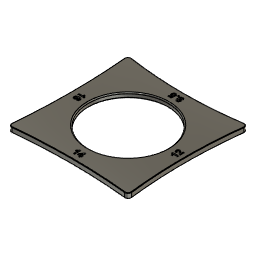
Radius Gauge (Autodesk Fusion 360 design; units mm, degrees)
Autodesk Fusion 360 part; units mm, degrees
note: some values were not read from the file. Set by a fixed rule: which sketch regions a step uses.
sketch "Sketch1" plane through (0, 0, 0) normal (0, 0, 1) x (1, 0, 0)
sketch "Sketch2" plane through (0, 0, 0) normal (0, 0, 1) x (1, 0, 0)
  line L0 (-38.1, 38.1) -> (38.1, 38.1)
  line L1 (38.1, 38.1) -> (38.1, -38.1)
  line L2 (38.1, -38.1) -> (-38.1, -38.1)
  line L3 (-38.1, -38.1) -> (-38.1, 38.1)
  line L4 (-38.1, 38.1) -> (38.1, -38.1) construction
  line L5 (38.1, 38.1) -> (-38.1, -38.1) construction
  circle A0 centre (0, 276.3731) radius 241.3
  circle A1 centre (340.5094, 0) radius 304.8
  circle A2 centre (0, -391.653) radius 355.6
  circle A3 centre (-442.7101, 0) radius 406.4
  line L6 (0, 38.1) -> (0, -38.1)
  line L7 (-36.3101, -0.008) -> (35.7094, -0.008)
  line L8 (5.8923, 32.385) -> (-5.8923, 32.385) construction
  line L9 (-5.8923, 32.385) -> (-5.8923, 28.3087) construction
  line L10 (-5.8923, 28.3087) -> (5.8923, 28.3087) construction
  line L11 (5.8923, 28.3087) -> (5.8923, 32.385) construction
  line L12 (34.2534, -4.0104, 1.27) -> (34.2534, 3.9945, 1.27) construction
  line L13 (34.2534, 3.9945, 1.27) -> (27.636, 3.9945, 1.27) construction
  line L14 (27.636, 3.9945, 1.27) -> (27.636, -4.0104, 1.27) construction
  line L15 (27.636, -4.0104, 1.27) -> (34.2534, -4.0104, 1.27) construction
  line L16 (-5.8677, -33.4751) -> (5.8677, -33.4751) construction
  line L17 (5.8677, -33.4751) -> (5.8677, -28.4153) construction
  line L18 (5.8677, -28.4153) -> (-5.8677, -28.4153) construction
  line L19 (-5.8677, -28.4153) -> (-5.8677, -33.4751) construction
  line L20 (-33.0497, 3.7941) -> (-33.0497, -3.81) construction
  line L21 (-33.0497, -3.81) -> (-28.6723, -3.81) construction
  line L22 (-28.6723, -3.81) -> (-28.6723, 3.7941) construction
  line L23 (-28.6723, 3.7941) -> (-33.0497, 3.7941) construction
  circle A4 centre (0, 0) radius 25.1447
  dimension "d1" = 76.2
  dimension "d2" = 76.2
  dimension "d3" = 482.6
  dimension "d4" = 609.6
  dimension "d5" = 711.2
  dimension "d6" = 812.8
  text T0 "9.5" font "Arial" height 3.81 bold align centre middle in box 11.7845 x 4.0763 at (5.8923, 32.385) x (-1, 0) y (0, -1) spacing 1
  text T1 "12" font "Arial" height 3.81 bold align centre middle in box 8.0049 x 6.6174 at (34.2534, -4.0104) x (0, 1) y (-1, 0) spacing 1
  text T2 "14" font "Arial" height 3.81 bold align centre middle in box 11.7354 x 5.0598 at (-5.8677, -33.4751) x (1, 0) y (0, 1) spacing 1
  text T3 "16" font "Arial" height 3.81 bold align centre middle in box 7.6041 x 4.3775 at (-33.0497, 3.7941) x (0, -1) y (1, 0) spacing 1
  constraint horizontal L0
  constraint perpendicular L0 L1
  constraint parallel L0 L2
  constraint parallel L1 L3
  constraint coincident L4 A4.centre
  constraint coincident L5 A4.centre
  constraint coincident A4.centre origin
  constraint coincident L0.start A0
  constraint coincident L0.end A0
  constraint coincident L0.end A1
  constraint coincident L1.end A1
  constraint coincident L1.end A2
  constraint coincident L2.end A2
  constraint coincident L0.start A3
  constraint coincident L2.end A3
  constraint midpoint L0 L6.start
  constraint midpoint L2 L6.end
  constraint coincident A3 L7.start
  constraint coincident A1 L7.end
  measures "d1" distance of L1.end L2.end
  measures "d2" distance of L0.end L1.end
  measures "d3" diameter of A0
  measures "d4" diameter of A1
  measures "d5" diameter of A2
  measures "d6" diameter of A3
extrude "Extrude1" add sketch "Sketch2" along normal blind 3.175 contours A0 A3 L6 L7 A4 | A2 A3 L6 L7 A4 | A0 A1 L6 L7 A4 | A1 A2 L6 L7 A4 | L6 L7 A4 | L6 L7 A4 | L6 L7 A4 | L6 L7 A4
emboss "Emboss1" depth -0.889 profiles "Sketch2" section 1 text T3 onto face at (-12.1034, -0.3293, 3.175)
emboss "Emboss2" depth -0.889 profiles "Sketch2" section 1 text T2 onto face at (6.5855, -16.8406, 3.175)
emboss "Emboss3" depth -0.889 profiles "Sketch2" section 1 text T1 onto face at (-4.6591, 2.6504, 3.175)
emboss "Emboss4" depth -0.889 profiles "Sketch2" section 1 text T0 onto face at (4.2989, 12.9497, 3.175)
fillet "Fillet1" radius 2.032 4 edges at (-38.1, 38.1, 1.5875) (38.1, 38.1, 1.5875) (38.1, -38.1, 1.5875) (-38.1, -38.1, 1.5875)
fillet "Fillet2" radius 0.254 16 edges at (-37.2338, 37.1747, 3.175) (-36.3101, -0.0637, 3.175) (-37.2799, -37.2685, 3.175) (-0.0386, -36.053, 3.175) (37.2236, -37.2396, 3.175) (35.7094, -0.0659, 3.175) (37.1738, 37.1419, 3.175) (-0.0409, 35.0731, 3.175) (37.1738, 37.1419, 0) (35.7094, -0.0659, 0) (37.2236, -37.2396, 0) (-0.0386, -36.053, 0) (-37.2799, -37.2685, 0) (-36.3101, -0.0637, 0) (-37.2338, 37.1747, 0) (-0.0409, 35.0731, 0)
extrude "Extrude2" cut sketch "Sketch2" along normal blind 40.64 and the other way blind 17.78 contours L6 L7 A4 | L6 L7 A4 | L6 L7 A4 | L6 L7 A4
fillet "Fillet3" radius 0.635 2 edges at (-23.4431, 9.0927, 3.175) (-23.4431, -9.0927, 0)
sketch "Sketch3" plane through (0, 0, 0) normal (0, 0, 1) x (1, 0, 0)
